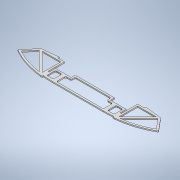
# Autodesk Inventor part: bulkhead_F1
Saved by Autodesk Inventor 2020.3 (Build 243373000, 373)
## iProperties
Created: 2020-05-22
Part Number: bulkhead_F1
Material: Generic
Document SubType Name: Modeling
Designer: kardo
Density: 1 g/cm^3
Appearance: Default
Mass: 4.97836 g
Surface Area: 76.7453 cm^2
Volume: 4.97836 cm^3
Author: kardo
Autodesk Inventor part; units mm, degrees
ref_plane "YZ Plane" through (0, 0, 0) normal (1, 0, 0) x (0, 1, 0)
ref_plane "XZ Plane" through (0, 0, 0) normal (0, 1, 0) x (-1, 0, 0)
ref_plane "XY Plane" through (0, 0, 0) normal (0, 0, 1) x (1, 0, 0)
derived "base_sketch.ipt"
sketch "bulkhead_F1" plane through (0, 56.1, 0) normal (0, 1, 0) x (-1, 0, 0)
  line L0 (19.176, 46.818) -> (62.322, 46.818)
  line L1 (-34.5168, 0) -> (-57.528, 27.54)
  line L2 (-11.5056, -2.4868) -> (-34.5168, 0)
  line L3 (-11.5056, 0) -> (-11.5056, -2.4868)
  line L4 (0, 0) -> (-11.5056, 0)
  line L5 (62.322, 46.818) -> (62.322, 13.2443)
  line L6 (28.764, 19.65) -> (28.764, 13.2443)
  line L7 (-39.7207, 4.4853) -> (-11.5056, 1.4361)
  line L8 (-11.5056, 1.4361) -> (-11.5056, 3.9229)
  line L9 (-11.5056, 3.9229) -> (0, 3.9229)
  line L10 (0, 3.9229) -> (0, 21.2783)
  line L11 (0, 21.2783) -> (28.764, 21.2783)
  line L12 (28.764, 21.2783) -> (28.764, 14.3875)
  line L13 (28.764, 14.3875) -> (62.322, 14.3875)
  line L14 (62.322, 43.0263) -> (19.176, 43.0263)
  line L15 (-57.528, 25.7972) -> (-39.7207, 4.4853)
  line L16 (0, 45.9) -> (0, 44.1572) construction
  line L17 (-19.176, 42.5952) -> (-19.176, 40.8524) construction
  line L18 (-38.352, 36.72) -> (-38.352, 34.9772) construction
  line L19 (-57.528, 27.54) -> (-57.528, 25.7972) construction
  line L20 (0, 19.65) -> (0, 0)
  line L21 (0, 44.1572) -> (0, 42.1083)
  line L22 (-57.528, 25.7972) -> (0, 35.7) construction
  spline S0 degree 4 poles (-57.528, 27.54) (-46.0483, 34.2051) (-30.6129, 40.5281) (-11.2214, 45.0414) (8.3201, 46.818) (15.5662, 46.818) (19.176, 46.818) knots 0 0 0 0 0 0.630279 0.815816 1 1 1 1 1
  spline S1 degree 3 poles (-57.528, 25.7972) (-39.18, 36.4663) (-19.6272, 41.8933) (0, 44.1572) knots 0 0 0 0 1 1 1 1
  spline S2 degree 2 poles (0, 42.1083) (9.5715, 43.0263) (19.176, 43.0263) knots 0 0 0 1 1 1
  point P0 (0, 14.3875)
  point P1 (0, 44.0613)
ref_plane "bulkhead_F1_plane" through (0, 56.1, 0) normal (0, 1, 0) x (-1, 0, 0)
sketch "Sketch2" plane through (0, 56.1, 0) normal (0, 1, 0) x (-1, 0, 0)
  spline S0 degree 2 poles (0, 42.1083) (9.5715, 43.0263) (19.176, 43.0263) knots 0 0 0 1 1 1 projected
  line L0 (62.322, 43.0263) -> (19.176, 43.0263) projected
  line L1 (62.322, 46.818) -> (62.322, 13.2443) projected
  line L2 (28.764, 14.3875) -> (62.322, 14.3875) projected
  line L3 (28.764, 21.2783) -> (28.764, 14.3875) projected
  line L4 (0, 21.2783) -> (28.764, 21.2783) projected
  line L5 (0, 3.9229) -> (0, 21.2783) projected
  line L6 (-11.5056, 3.9229) -> (0, 3.9229) projected
  line L7 (-11.5056, 1.4361) -> (-11.5056, 3.9229) projected
  line L8 (-39.7207, 4.4853) -> (-11.5056, 1.4361) projected
  line L9 (-57.528, 25.7972) -> (-39.7207, 4.4853) projected
  spline S1 degree 3 poles (-57.528, 25.7972) (-39.18, 36.4663) (-19.6272, 41.8933) (0, 44.1572) knots 0 0 0 0 1 1 1 1 projected
  line L10 (-52.9133, 24.9531) -> (-38.8771, 8.1545)
  line L11 (-38.8771, 8.1545) -> (-6.7834, 40.2089)
  line L12 (-34.4499, 6.9229) -> (-3, 38.3342)
  line L13 (-3, 38.3342) -> (-3, 6.9229)
  line L14 (-3, 6.9229) -> (-34.4499, 6.9229)
  line L15 (0, 21.2783) -> (0, 31.6933)
  line L16 (0, 31.6933) -> (2, 31.6933)
  line L17 (2, 31.6933) -> (2, 21.2783)
  line L18 (16.176, 37.1083) -> (16.176, 26.2783)
  line L19 (14.176, 24.2783) -> (7, 24.2783)
  line L20 (5, 26.2783) -> (5, 37.1083)
  line L21 (7, 39.1083) -> (14.176, 39.1083)
  line L22 (22.176, 38.0263) -> (22.176, 26.2783)
  line L23 (24.176, 24.2783) -> (29.764, 24.2783)
  line L24 (31.764, 22.2783) -> (31.764, 19.3875)
  line L25 (33.764, 17.3875) -> (62.322, 17.3875)
  line L26 (24.176, 40.0263) -> (62.322, 40.0263)
  spline S2 degree 2 poles (-52.9133, 24.9531) (-31.1706, 36.5792) (-6.7834, 40.2089) knots 0 0 0 1 1 1
  line L27 (-6.7834, 40.2089) -> (-7.2485, 43.1726) construction
  line L28 (-30.5095, 34.5801) -> (-31.4398, 37.4322) construction
  line L29 (-52.9133, 24.9531) -> (-54.3489, 27.5873) construction
  line L30 (-52.9133, 24.9531) -> (-30.5095, 34.5801) construction
  line L31 (-30.5095, 34.5801) -> (-6.7834, 40.2089) construction
  line L32 (-39.7207, 4.4853) -> (0, 44.1572) construction
  arc A0 (14.176, 24.2783) -> (16.176, 26.2783) centre (14.176, 26.2783) ccw
  arc A1 (5, 26.2783) -> (7, 24.2783) centre (7, 26.2783) ccw
  arc A2 (7, 39.1083) -> (5, 37.1083) centre (7, 37.1083) ccw
  arc A3 (16.176, 37.1083) -> (14.176, 39.1083) centre (14.176, 37.1083) ccw
  arc A4 (24.176, 40.0263) -> (22.176, 38.0263) centre (24.176, 38.0263) ccw
  arc A5 (22.176, 26.2783) -> (24.176, 24.2783) centre (24.176, 26.2783) ccw
  arc A6 (31.764, 22.2783) -> (29.764, 24.2783) centre (29.764, 22.2783) ccw
  arc A7 (31.764, 19.3875) -> (33.764, 17.3875) centre (33.764, 19.3875) ccw
  line L33 (62.322, 43.0263) -> (62.322, 14.3875)
  line L34 (0, 44.1572) -> (0, 42.1083) projected
  line L35 (0, 44.1572) -> (2, 44.1572)
  line L36 (2, 44.1572) -> (2, 42.29)
  line L37 (0, 42.1083) -> (0, 31.6933) construction
  point P0 (0, 0)
  point P1 (0, 44.0613)
  dimension "d1" = 3
  dimension "d2" = 3
  dimension "d3" = 3
  dimension "d4" = 4
  dimension "d5" = 2
  dimension "d6" = 3
  dimension "d7" = 3
  dimension "d8" = 3
  dimension "d9" = 3
  dimension "d10" = 3
  dimension "d11" = 3
  dimension "d12" = 3
  dimension "d13" = 3
  dimension "d14" = 3
  dimension "d15" = 3
  dimension "d16" = 2
  constraints: 54 end point, 16 point on circle, 16 tangent, 9 parallel, 8 centre point, 7 equal radius, 7 vertical, 4 equal length, 3 horizontal, 3 point on line, 2 perpendicular, 1 collinear, 11 other
  measures "d1" distance between parallel lines of L6 L14
  measures "d2" distance between parallel lines of L5 L13
  measures "d3" distance between parallel lines of L9 L10
  measures "d4" distance between parallel lines of L12 L11
  measures "d5" distance between parallel lines of L17 L15
  measures "d6" distance between parallel lines of L20 L17
  measures "d7" distance from line of L34.end L21
  measures "d8" distance between parallel lines of L4 L19
  measures "d9" distance from line of L0.end L18
  measures "d10" distance from line of L0.end L22
  measures "d11" distance between parallel lines of L2 L25
  measures "d12" distance between parallel lines of L3 L24
  measures "d13" distance between parallel lines of L4 L23
  measures "d14" distance between parallel lines of L0 L26
  measures "d15" distance of L10.start L29.end
  measures "d16" radius of A0
extrude "Extrusion1" add sketch "Sketch2" along normal blind 2 contours L34 L35 L36 S0 | S0 L0 L1 L26 A4 L22 A5 L23 A6 L24 A7 L25 L2 L3 L4 L17 L16 L15 L5 L6 L7 L8 L9 S1 L34
mirror "Mirror1" about plane through (-62.322, 56.1, 14.3875) normal (-1, 0, 0) of "Extrusion1"
equation "\"d5\" = stringer_thickness"
equation "\"d17\" = bulkhead_thickness"
equation "\"stringer_thickness\" = 2"
equation "\"bulkhead_thickness\" = 2"
body "Solid1"
